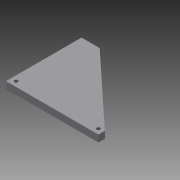
# Autodesk Inventor part: BallGuidePlyRight
Saved by Autodesk Inventor 2014 (Build 180170000, 170)
## iProperties
Created: 2016-02-08
Part Number: BallGuidePlyRight
Material: Generic
Document SubType Name: Modeling
Designer: choices
Density: 1 g/cm^3
Appearance: Default
Author: choices
Autodesk Inventor part; units mm, degrees
ref_plane "YZ Plane" through (0, 0, 0) normal (1, 0, 0) x (0, 1, 0)
ref_plane "XZ Plane" through (0, 0, 0) normal (0, 1, 0) x (-1, 0, 0)
ref_plane "XY Plane" through (0, 0, 0) normal (0, 0, 1) x (1, 0, 0)
sketch "Sketch1" plane through (0, 0, 0) normal (0, 1, 0) x (-1, 0, 0)
  line L0 (-111.8414, 23.1497) -> (72.3086, 23.1497)
  line L1 (72.3086, 23.1497) -> (72.3086, -148.2749)
  line L2 (72.3086, -148.2749) -> (-111.8414, 23.1497)
  circle A0 centre (62.7836, 13.6247) radius 3.3528
  circle A1 centre (-89.6164, 13.6247) radius 3.3566
  line L3 (-99.1414, 23.1497) -> (-99.1414, 11.3273)
  line L4 (38.6383, -116.9313) -> (72.3086, -116.9313)
  point P0 (0, 0)
  dimension "d0" = 184.15
  dimension "d1" = 171.4246
  dimension "d2" = 6.7056
  dimension "d3" = 9.525
  dimension "d4" = 6.7132
  dimension "d5" = 152.4
  dimension "d8" = 12.7
  dimension "d9" = 9.525
  dimension "d10" = 140.081
  constraints: 10 end point, 4 point on line, 2 centre point, 2 perpendicular, 1 horizontal, 1 parallel
  measures "d0" distance of L0.start L0.end
  measures "d1" distance of L0.end L1.end
  measures "d2" diameter of A0
  measures "d3" distance from line of L0 A0.centre
  measures "d4" diameter of A1
  measures "d5" distance of A0.centre A1.centre
  measures "d8" distance from line of L3 L0.start
  measures "d9" distance from line of L1 A0.centre
  measures "d10" distance between parallel lines of L0 L4
extrude "Extrusion1" add sketch "Sketch1" along normal blind 12.7 contours L0 L1 L4 L2 L3
body "Solid1"
